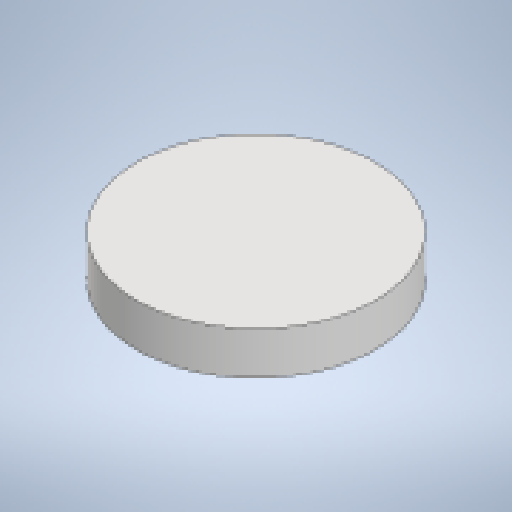
# Autodesk Inventor part: 8mm axle mount
Saved by Autodesk Inventor 2025 (Build 290162000, 162)
## iProperties
Created: 2025-04-20
Part Number: 8mm axle mount
Material: 一般
Document SubType Name: Modeling
Designer: gavin
Density: 1 g/cm^3
Appearance: 預設
Author: gavin
Autodesk Inventor part; units mm, degrees
ref_plane "YZ Plane" through (0, 0, 0) normal (1, 0, 0) x (0, 1, 0)
ref_plane "XZ Plane" through (0, 0, 0) normal (0, 1, 0) x (-1, 0, 0)
ref_plane "XY Plane" through (0, 0, 0) normal (0, 0, 1) x (1, 0, 0)
sketch "草圖1" plane through (0, 0, 0) normal (0, 1, 0) x (-1, 0, 0)
  circle A0 centre (0, 0) radius 14
  circle A1 centre (0, 0) radius 10
  circle A2 centre (10, 0) radius 1.75
  circle A3 centre (0, 10) radius 1.75
  circle A4 centre (-10, 0) radius 1.75
  circle A5 centre (0, -10) radius 1.75
  dimension "d3" = 20
  dimension "d0" = 28
  dimension "d4" = 3.5
  dimension "d7" = 360
  constraints: 5 centre point, 2 coincident, 1 horizontal alignment, 11 other
  measures "d0" diameter of A0
  measures "d4" diameter of A2
extrude "擠出1" add sketch "草圖1" along normal blind 5 contours A0 | A2 A1 A5 A4 A3
sketch "草圖2" plane through (0, 5, 0) normal (0, 1, 0) x (1, 0, 0)
  circle A0 centre (0, 0) radius 6
  dimension "d9" = 12
  constraints: 1 centre point, 1 coincident
  measures "d9" diameter of A0
extrude "擠出2" add sketch "草圖2" along normal blind 11
sketch "草圖3" plane through (0, 16, 0) normal (0, 1, 0) x (1, 0, 0)
  circle A0 centre (0, 0) radius 4
  dimension "d12" = 8
  constraints: 1 centre point, 1 coincident
  measures "d12" diameter of A0
extrude "擠出3" cut sketch "草圖3" against normal through all
